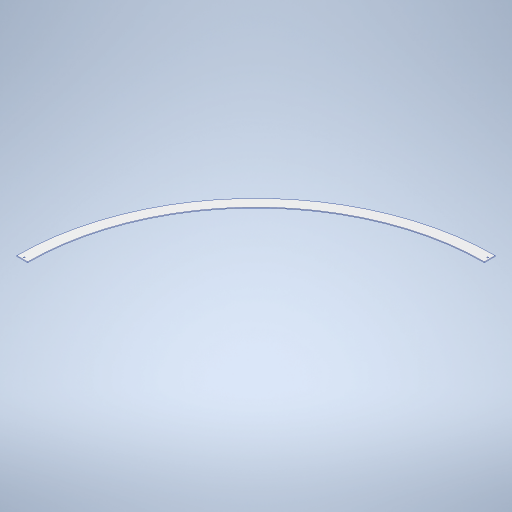
# Autodesk Inventor part: Arco médio
Saved by Autodesk Inventor 2024 (Build 280153000, 153)
## iProperties
Created: 2024-05-05
Part Number: Arco médio
Material: Alumínio 6061
Document SubType Name: Modeling
Designer: mathe
Density: 2.7 g/cm^3
Appearance: Alumínio - Plano
Author: mathe
Autodesk Inventor part; units mm, degrees
ref_plane "YZ Plane" through (0, 0, 0) normal (1, 0, 0) x (0, 1, 0)
ref_plane "XZ Plane" through (0, 0, 0) normal (0, 1, 0) x (-1, 0, 0)
ref_plane "XY Plane" through (0, 0, 0) normal (0, 0, 1) x (1, 0, 0)
sketch "Esboço1" plane through (0, 0, 0) normal (0, 1, 0) x (-1, 0, 0)
  arc A0 (-491.7313, -306.4749) -> (358.2687, 543.5251) centre (-491.7313, 543.5251) ccw
  arc A1 (-491.7313, -346.4749) -> (398.2687, 543.5251) centre (-491.7313, 543.5251) ccw
  line L0 (358.2687, 543.5251) -> (398.2687, 543.5251)
  line L1 (-491.7313, -306.4749) -> (-491.7313, -346.4749)
  point P0 (0, 0)
  dimension "d0" = 850
  dimension "d1" = 890
  constraints: 4 end point, 4 point on circle, 2 centre point, 2 coincident, 1 horizontal, 1 perpendicular
  measures "d0" radius of A0
  measures "d1" radius of A1
extrude "Extrusão1" add sketch "Esboço1" along normal blind 3
sketch "Esboço2" plane through (0, 3, 0) normal (0, 1, 0) x (1, 0, 0)
  circle A0 centre (-378.2687, -536.0251) radius 2.5
  circle A1 centre (484.2313, 326.4749) radius 2.5
  line L0 (491.7313, 306.4749) -> (491.7313, 346.4749) projected
  line L1 (-398.2687, -543.5251) -> (-358.2687, -543.5251) projected
  point P0 (0, 0)
  dimension "d16" = 5
  dimension "d17" = 5
  dimension "d18" = 7.5
  dimension "d19" = 20
  dimension "d20" = 7.5
  dimension "d21" = 20
  constraints: 2 centre point
  measures "d16" diameter of A0
  measures "d17" diameter of A1
  measures "d18" distance from line of L0 A1.centre
  measures "d19" vertical distance of L0.end A1.centre
  measures "d20" distance from line of L1 A0.centre
  measures "d21" horizontal distance of L1.start A0.centre
hole "Furo1" at (-378.2687, 3, 536.0251) at (484.2313, 3, -326.4749) direction (0, -1, 0) diameter 5 end through all
